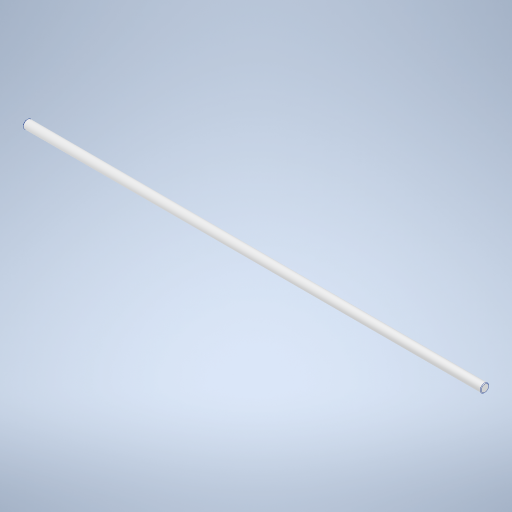
# Autodesk Inventor part: 8mm Rod ~44cm
Saved by Autodesk Inventor 2024 (Build 280153000, 153)
## iProperties
Created: 2023-12-05
Part Number: 8mm Rod ~44cm
Material: Aluminum 6061
Document SubType Name: Modeling
Designer: 18179
Density: 2.7 g/cm^3
Appearance: Aluminum - Flat
Author: 18179
Autodesk Inventor part; units mm, degrees
ref_plane "YZ Plane" through (0, 0, 0) normal (1, 0, 0) x (0, 1, 0)
ref_plane "XZ Plane" through (0, 0, 0) normal (0, 1, 0) x (-1, 0, 0)
ref_plane "XY Plane" through (0, 0, 0) normal (0, 0, 1) x (1, 0, 0)
sketch "Sketch1" plane through (0, 0, 0) normal (1, 0, 0) x (0, 1, 0)
  circle A0 centre (0, 0) radius 4
  dimension "d0" = 8
  constraints: 1 centre point, 1 coincident
  measures "d0" diameter of A0
extrude "Extrusion1" add sketch "Sketch1" along normal blind 437.5
chamfer "Chamfer1" distance 0.508 angle 45 2 edges at (0, -4, 0) (437.5, -4, 0)
body "Solid1"
